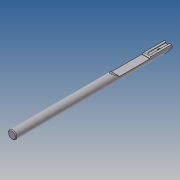
# Autodesk Inventor part: J008040 NEUROPIXELS GEN 2 DOVE TAIL PROBE HOLDER Rev -
Saved by Autodesk Inventor 2018.3 (Build 223284000, 284)
## iProperties
Created: 2017-01-23
Material: ALUMINUM, 7075-T651
Vendor: HHMI: JRC - ID&F
Document SubType Name: Modeling
Designer: ARNOLDJ
Density: 2.81 g/cm^3
Appearance: Metal-AL-6061 (Machined)
Description: NEUROPIXELS GEN 2DOVE TAIL PROBE HOLDER
Part Number: J008040 NEUROPIXELS GEN 2 DOVE TAIL PROBE HOLDER Rev -
RuleStatus: InUse
AfterDocSave0: file://Part Number Cleaner
LAB/DEPT: APIG (SHARED RESOURCE)
SURFACE ROUGHNESS: 32 Ra
DESIGN DEPARTMENT: HHMI: JRC - ID&F
SPECIAL FINISH: NONE
ALTERED ITEM PART NUMBER: N/A
ALTERED ITEM VENDOR: N/A
ALTERED ITEM DESCRIPTION: N/A
Author: ARNOLDJ
Revision Number: 0
Autodesk Inventor part; units mm, degrees
ref_plane "YZ Plane" through (0, 0, 0) normal (1, 0, 0) x (0, 1, 0)
ref_plane "XZ Plane" through (0, 0, 0) normal (0, 1, 0) x (-1, 0, 0)
ref_plane "XY Plane" through (0, 0, 0) normal (0, 0, 1) x (1, 0, 0)
sketch "Sketch1" plane through (0, 0, 0) normal (0, 0, 1) x (1, 0, 0)
  circle A0 centre (0, 0) radius 2.00025
  dimension "d0" = 4.0005
  constraints: 1 centre point, 1 coincident
  measures "d0" diameter of A0
extrude "Extrusion1" add sketch "Sketch1" along normal blind 75
sketch "Sketch2" plane through (0, 0, 0) normal (0, 0, 1) x (1, 0, 0)
  circle A0 centre (0, 0) radius 2.00025
  line L0 (1.353027, 1.4732) -> (-1.353027, 1.4732)
  line L1 (0, 2.80035) -> (0, -2.80035)
  line L2 (-2.80035, 0) -> (2.80035, 0)
  line L3 (1.723004, 1.016) -> (-1.723004, 1.016)
  line L4 (0.7112, 1.016) -> (1.18047, 0.2032)
  line L5 (1.18047, 0.2032) -> (-1.18047, 0.2032)
  line L6 (-1.18047, 0.2032) -> (-0.7112, 1.016)
  line L7 (0, 0) -> (0, 2.00025)
  dimension "d6" = 1.016
  dimension "d9" = 60
  dimension "d10" = 1.4224
  dimension "d11" = 0.8128
  dimension "d40" = 0.4572
  constraints: 12 end point, 5 point on circle, 3 horizontal, 3 point on line, 1 equal length, 1 other
  measures "d6" distance between parallel lines of L3 L2
  measures "d9" angle of L5 L4
  measures "d10" distance of L6.end L4.start
  measures "d11" distance between parallel lines of L5 L3
  measures "d40" distance between parallel lines of L3 L0
extrude "Extrusion3" cut sketch "Sketch2" along normal blind 9.525 contours L3 L1 L0 A0 | L1 L3 A0 L0
extrude "Extrusion4" cut sketch "Sketch2" along normal blind 8.763 contours L4 L5 L1 L3 | L5 L6 L3 L1
sketch "Sketch3" plane through (-1.18047, 0.2032, 9.525) normal (0, 1, 0) x (1, 0, 0)
  line L0 (0, 9.525) -> (2.360941, 9.525)
  line L1 (1.18047, 24.525) -> (1.18047, -80.475)
  point P0 (1.18047, 9.525)
  point P1 (1.18047, 5.334)
  dimension "d14" = 4.191
  constraints: 1 point on line
  measures "d14" distance from line of point (1.18, 5.334) L0
hole "Hole1" at (0, 0.2032, 4.191) direction (0, -1, 0) diameter 1.2192 end through all thread size "M1.6x0.35" class "6H" standard "ANSI Metric M Profile"
sketch "Sketch4" plane through (0, 0, 0) normal (1, 0, 0) x (0, 1, 0)
  line L0 (0, 120) -> (0, -20)
  line L1 (-2.00025, 0) -> (-2.00025, 75)
  line L2 (0, 0) -> (-2.00025, 3.464535)
  line L3 (-2.00025, 3.464535) -> (-2.00025, 0)
  line L4 (-2.00025, 0) -> (0, 0)
  dimension "d23" = 30
  constraints: 6 end point, 1 collinear, 1 perpendicular, 1 point on line
  measures "d23" angle of L0 L2
extrude "Extrusion5" cut sketch "Sketch4" along normal mid plane 12.7
chamfer "Chamfer1" distance 0.254 distance2 0.381 1 edges at (-0.9458, 0.6096, 0) measured on face at (-1.2049, 0.7451, 0)
chamfer "Chamfer2" distance 0.254 distance2 0.381 1 edges at (0.9458, 0.6096, 0) measured on face at (1.2049, 0.7451, 0)
chamfer "Chamfer3" distance 0.381 angle 45 1 edges at (-2.0003, 0, 75)
extrude "Extrusion7" cut sketch "Sketch2" along normal blind 25.4 contours L3 L1 L0 A0 | L0 L1 A0 | L1 L0 A0 | L1 L3 A0 L0
sketch "Sketch6" plane through (-0.7112, 1.016, 9.525) normal (0, 1, 0) x (1, 0, 0)
  line L0 (-1.011804, -15.875) -> (2.434204, -15.875)
  line L1 (0.7112, 24.525) -> (0.7112, -80.475)
  line L2 (6.9342, 9.525) -> (-5.5118, 9.525)
  line L3 (5.1562, -1.143) -> (-3.7338, -1.143)
  line L4 (-3.7338, -1.143) -> (-3.7338, -15.875)
  line L5 (-3.7338, -15.875) -> (5.1562, -15.875)
  line L6 (5.1562, -15.875) -> (5.1562, -1.143)
  line L7 (5.1562, -1.143) -> (-3.7338, -15.875) construction
  line L8 (-3.7338, -1.143) -> (5.1562, -15.875) construction
  point P0 (0.7112, 9.525)
  point P1 (0.7112, -8.509)
  dimension "d43" = 0
  dimension "d45" = 8.89
  dimension "d68" = 10.668
  dimension "d69" = 14.732
  constraints: 12 end point, 2 midpoint, 2 parallel, 1 horizontal, 1 perpendicular, 1 point on line
  measures "d43" distance between parallel lines of L5 L0
  measures "d45" distance of L3.start L3.end
  measures "d68" distance between parallel lines of L2 L3
  measures "d69" distance of L3.end L4.end
extrude "Extrusion8" cut sketch "Sketch6" against normal blind 0.508
sketch "Sketch11" plane through (0, 0, 0) normal (1, 0, 0) x (0, 1, 0)
  line L0 (0.508, 10.668) -> (0.508, 25.4)
  line L1 (2.00025, 25.4) -> (2.00025, 74.619)
  line L2 (0.635, 25.4) -> (2.00025, 27.764682)
  line L3 (0.508, 10.668) -> (1.016, 10.668)
  line L4 (-0.40005, 0) -> (2.4003, 0)
  line L5 (0.635, 10.668) -> (1.016, 10.008089)
  line L6 (1.016, 10.008089) -> (1.016, 10.668)
  line L7 (0.635, 10.668) -> (1.016, 10.668)
  line L8 (2.00025, 27.764682) -> (2.00025, 25.4)
  line L9 (2.00025, 25.4) -> (0.508, 25.4)
  line L10 (0.635, 25.4) -> (2.00025, 25.4)
  point P0 (0, 0)
  dimension "d56" = 0.127
  dimension "d57" = 10.668
  dimension "d58" = 0.127
  dimension "d59" = 30
  dimension "d64" = 30
  constraints: 12 end point, 2 horizontal, 2 vertical, 1 point on line
  measures "d56" distance from line of L0 L2.start
  measures "d57" distance between parallel lines of L4 L3
  measures "d58" distance from line of L5.start L0
  measures "d59" angle of L5 L6
  measures "d64" angle of L1 L2
extrude "Extrusion10" cut sketch "Sketch11" along normal mid plane 6.35
sketch "Sketch12" plane through (-1.473764, 0.2032, 0) normal (0, 1, 0) x (1, 0, 0)
  circle A0 centre (1.473764, -4.191) radius 0.6096
  circle A1 centre (1.473764, -4.191) radius 0.8
  circle A2 centre (1.473764, -4.191) radius 0.7
  point P0 (1.473764, 0)
  dimension "d65" = 1.6
  dimension "d66" = 1.4
  constraints: 2 centre point, 2 coincident
  measures "d65" diameter of A1
  measures "d66" diameter of A2
sketch "Sketch14" plane through (0, 0, 8.763) normal (0, 0, -1) x (-1, 0, 0)
  line L0 (0.7112, 1.016) -> (1.18047, 0.2032)
  line L1 (-1.473764, 0.2032) -> (1.473764, 0.2032)
  line L2 (0.7112, 1.016) -> (0.7112, 0.2032)
  line L3 (1.18047, 0.2032) -> (-1.18047, 0.2032)
  line L4 (0.7112, 0.2032) -> (1.18047, 0.2032)
  line L5 (0, -2.80035) -> (0, 2.80035)
  line L6 (0, 0.2032) -> (0, 1.016)
  line L7 (0.7112, 1.016) -> (0, 1.016)
  line L8 (0, 1.016) -> (0, 0.2032)
  line L9 (0, 0.2032) -> (0.7112, 0.2032)
  line L10 (0.7112, 0.2032) -> (0.7112, 1.016)
  point P0 (0, 0)
  constraints: 14 end point, 3 point on line, 2 parallel, 2 perpendicular, 1 collinear, 1 horizontal, 1 midpoint
revolve "Revolution1" cut sketch "Sketch14" angle 360 about axis through (0, 0, 8.763) along (0, 1, 0)
body "Solid1"
